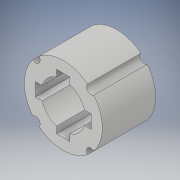
# Autodesk Inventor part: shaft_spacer
Saved by Autodesk Inventor 2019 (Build 230136000, 136)
## iProperties
Created: 2019-11-07
Part Number: shaft_spacer
Material: Generic
Document SubType Name: Modeling
Designer: luua
Density: 1 g/cm^3
Appearance: Default
Author: luua
Autodesk Inventor part; units mm, degrees
ref_plane "YZ Plane" through (0, 0, 0) normal (1, 0, 0) x (0, 1, 0)
ref_plane "XZ Plane" through (0, 0, 0) normal (0, 1, 0) x (-1, 0, 0)
ref_plane "XY Plane" through (0, 0, 0) normal (0, 0, 1) x (1, 0, 0)
sketch "Sketch1" plane through (0, 0, 0) normal (0, 0, 1) x (1, 0, 0)
  line L0 (-17.5, 0) -> (17.5, 0) construction
  line L1 (0, 12.4072) -> (0, -12.4072) construction
  line L2 (-12.5394, 0) -> (-12.5394, 3)
  line L3 (-12.5394, 3) -> (-9.5394, 3)
  line L4 (0, 12.5394) -> (-3, 12.5394)
  line L5 (-3, 12.5394) -> (-3, 9.5394)
  circle A0 centre (0, 0) radius 10 construction
  circle A1 centre (0, 0) radius 17.5 construction
  arc A2 (-3, 9.5394) -> (-9.5394, 3) centre (0, 0) ccw
  arc A3 (-13.7055, 10.8817) -> (-17.5, 0) centre (0, 0) ccw
  line L6 (0, 0) -> (-12.3744, 12.3744) construction
  line L7 (0, 0) -> (17.5, 0) construction
  arc A4 (0, 17.5) -> (-10.8817, 13.7055) centre (0, 0) ccw
  arc A5 (-13.7055, 10.8817) -> (-10.8817, 13.7055) centre (-12.3744, 12.3744) ccw
  line L8 (12.5394, 3) -> (9.5394, 3)
  line L9 (3, 12.5394) -> (3, 9.5394)
  arc A6 (9.5394, 3) -> (3, 9.5394) centre (0, 0) ccw
  arc A7 (10.8817, 13.7055) -> (13.7055, 10.8817) centre (12.3744, 12.3744) ccw
  line L10 (12.5394, 0) -> (12.5394, 3)
  line L11 (0, 12.5394) -> (3, 12.5394)
  arc A8 (17.5, 0) -> (13.7055, 10.8817) centre (0, 0) ccw
  arc A9 (10.8817, 13.7055) -> (0, 17.5) centre (0, 0) ccw
  line L12 (-12.5394, 0) -> (-12.5394, -3)
  line L13 (-12.5394, -3) -> (-9.5394, -3)
  line L14 (-3, -12.5394) -> (-3, -9.5394)
  arc A10 (-9.5394, -3) -> (-3, -9.5394) centre (0, 0) ccw
  arc A11 (-17.5, 0) -> (-13.7055, -10.8817) centre (0, 0) ccw
  arc A12 (-10.8817, -13.7055) -> (-13.7055, -10.8817) centre (-12.3744, -12.3744) ccw
  line L15 (0, -12.5394) -> (-3, -12.5394)
  line L16 (3, -12.5394) -> (3, -9.5394)
  arc A13 (3, -9.5394) -> (9.5394, -3) centre (0, 0) ccw
  line L17 (12.5394, -3) -> (9.5394, -3)
  line L18 (0, -12.5394) -> (3, -12.5394)
  line L19 (12.5394, 0) -> (12.5394, -3)
  arc A14 (13.7055, -10.8817) -> (17.5, 0) centre (0, 0) ccw
  arc A15 (0, -17.5) -> (10.8817, -13.7055) centre (0, 0) ccw
  arc A16 (13.7055, -10.8817) -> (10.8817, -13.7055) centre (12.3744, -12.3744) ccw
  arc A17 (-10.8817, -13.7055) -> (0, -17.5) centre (0, 0) ccw
  point P0 (12.3744, 12.3744)
  point P1 (-12.3744, -12.3744)
  point P2 (12.3744, -12.3744)
  dimension "d2" = 35
  dimension "d0" = 3
  dimension "d1" = 20
  dimension "d3" = 135
  dimension "d4" = 2
  constraints: 40 end point, 40 point on circle, 30 symmetric about line, 17 centre point, 10 coincident, 4 equal length, 3 horizontal, 2 midpoint, 2 perpendicular, 2 point on line, 2 vertical, 1 concentric, 17 other
  measures "d0" distance of L2.start L2.end
  measures "d1" diameter of A0
  measures "d3" angle of L7 L6
  measures "d4" radius of A5
extrude "Extrusion1" add sketch "Sketch1" along normal blind 24
body "Solid1"
